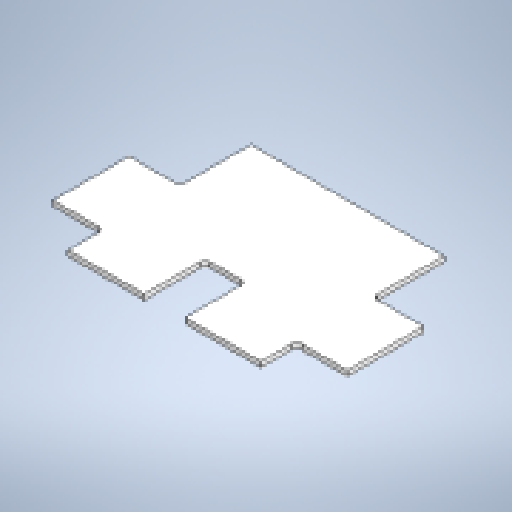
# Autodesk Inventor part: Bottom Plate
Saved by Autodesk Inventor 2023.2 (Build 272271000, 271)
## iProperties
Created: 2023-11-13
Part Number: Bottom Plate
Material: UHMW, White
Document SubType Name: Modeling
Designer: Nathan Cai
Density: 0.94 g/cm^3
Appearance: Smooth - White
Mass: 47.3333 g
Surface Area: 338.306 cm^2
Volume: 50.3546 cm^3
Author: Nathan Cai
Autodesk Inventor part; units mm, degrees
ref_plane "YZ Plane" through (0, 0, 0) normal (1, 0, 0) x (0, 1, 0)
ref_plane "XZ Plane" through (0, 0, 0) normal (0, 1, 0) x (-1, 0, 0)
ref_plane "XY Plane" through (0, 0, 0) normal (0, 0, 1) x (1, 0, 0)
sketch "Sketch1" plane through (0, 0, 0) normal (0, 1, 0) x (-1, 0, 0)
  line L0 (60.325, 57.15) -> (-60.325, 57.15)
  line L1 (-60.325, 57.15) -> (-60.325, -57.15)
  line L2 (-60.325, -57.15) -> (60.325, -57.15)
  line L3 (60.325, -57.15) -> (60.325, 57.15)
  line L4 (60.325, 57.15) -> (-60.325, -57.15) construction
  line L5 (-60.325, 57.15) -> (60.325, -57.15) construction
  line L6 (12.7, 95.25) -> (-12.7, 95.25)
  line L7 (-12.7, 95.25) -> (-12.7, 19.05)
  line L8 (-12.7, 19.05) -> (12.7, 19.05)
  line L9 (12.7, 19.05) -> (12.7, 95.25)
  line L10 (12.7, 95.25) -> (-12.7, 19.05) construction
  line L11 (-12.7, 95.25) -> (12.7, 19.05) construction
  line L12 (0, 57.15) -> (0, -57.15) construction
  line L13 (-92.075, 34.925) -> (92.075, 34.925)
  line L14 (92.075, 34.925) -> (92.075, -12.7)
  line L15 (92.075, -12.7) -> (-92.075, -12.7)
  line L16 (-92.075, -12.7) -> (-92.075, 34.925)
  line L17 (-92.075, 34.925) -> (92.075, -12.7) construction
  line L18 (92.075, 34.925) -> (-92.075, -12.7) construction
  point P0 (0, 0)
  point P1 (12.7, 57.15)
  point P2 (-12.7, 57.15)
  point P3 (0, 11.1125)
  point P4 (60.325, 34.925)
  point P5 (60.325, -12.7)
  point P6 (-60.325, -12.7)
  point P7 (-60.325, 34.925)
  dimension "d0" = 120.65
  dimension "d1" = 114.3
  dimension "d2" = 25.4
  dimension "d3" = 76.2
  dimension "d6" = 184.15
  dimension "d7" = 22.225
  dimension "d8" = 44.45
  constraints: 38 end point, 8 midpoint, 6 parallel, 3 horizontal, 3 perpendicular, 1 point on line
  measures "d0" distance of L2.end L1.end
  measures "d1" distance of L1.end L0.end
  measures "d2" distance of L8.end L7.end
  measures "d3" distance of L7.end L6.end
  measures "d6" distance of L14.end L15.end
  measures "d7" distance between parallel lines of L0 L13
  measures "d8" distance between parallel lines of L2 L15
extrude "Extrusion1" add sketch "Sketch1" along normal blind 3.175 contours L3 L13 L9 L0 | L13 L14 L15 L3 | L3 L15 L1 L13 L7 L8 L9 | L7 L13 L1 L0 | L3 L2 L1 L15 | L15 L16 L13 L1
fillet "Fillet1" radius 3.175 6 edges at (60.325, 1.5875, 34.925) (60.325, 1.5875, -12.7) (-12.7, 1.5875, 19.05) (12.7, 1.5875, 19.05) (-60.325, 1.5875, 34.925) (-60.325, 1.5875, -12.7)
body "Solid1"
